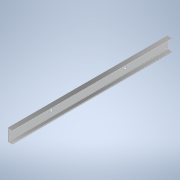
# Autodesk Inventor part: NASA-20-OP-01
Saved by Autodesk Inventor 2020 (Build 240168000, 168)
## iProperties
Created: 2019-09-07
Part Number: NASA-20-OP-01
Material: Aluminum 6061
Document SubType Name: Modeling
Designer: Rick Szalay
Density: 2.7 g/cm^3
Appearance: Aluminum - Flat
Author: Rick Szalay
Autodesk Inventor part; units mm, degrees
ref_plane "YZ Plane" through (0, 0, 0) normal (1, 0, 0) x (0, 1, 0)
ref_plane "XZ Plane" through (0, 0, 0) normal (0, 1, 0) x (-1, 0, 0)
ref_plane "XY Plane" through (0, 0, 0) normal (0, 0, 1) x (1, 0, 0)
sketch "Sketch1" plane through (0, 0, 0) normal (0, 0, 1) x (1, 0, 0)
  line L0 (0, 25.4) -> (0, -25.4)
  line L1 (0, -25.4) -> (19.05, -25.4)
  line L2 (0, 25.4) -> (19.05, 25.4)
  line L3 (19.05, 25.4) -> (19.05, 22.225)
  line L4 (19.05, 22.225) -> (3.048, 22.225)
  line L5 (3.048, 22.225) -> (3.048, -22.225)
  line L6 (3.048, -22.225) -> (19.05, -22.225)
  line L7 (19.05, -22.225) -> (19.05, -25.4)
  point P0 (0, 0)
  point P1 (0, 0)
  dimension "d0" = 50.8
  dimension "d1" = 19.05
  dimension "d2" = 3.175
  dimension "d3" = 16.002
  constraints: 16 end point, 5 perpendicular, 2 equal length, 2 vertical, 1 coincident, 1 horizontal, 1 midpoint, 1 point on line
  measures "d0" distance of L0.start L0.end
  measures "d1" distance of L0.start L2.end
  measures "d2" distance between parallel lines of L4 L2
  measures "d3" distance between parallel lines of L5 L7
extrude "Extrusion1" add sketch "Sketch1" along normal mid plane 660.4
fillet "Fillet1" radius 1.5875 4 edges at (3.048, 22.225, 0) (3.048, -22.225, 0) (19.05, -22.225, 0) (19.05, 22.225, 0)
sketch "Sketch2" plane through (3.048, -20.6375, -330.2) normal (1, 0, 0) x (0, 0, -1)
  point P0 (-330.2, 20.6375)
  point P1 (-177.8, 20.6375)
  point P2 (-482.6, 20.6375)
  dimension "d7" = 304.8
  dimension "d8" = 152.4
  constraints: 2 horizontal alignment
  measures "d7" distance of point (-482.6, 20.637) point (-177.8, 20.637)
  measures "d8" distance of point (-177.8, 20.637) point (-330.2, 20.637)
hole "Hole1" at (3.048, 0, -152.4) at (3.048, 0, 152.4) direction (-1, 0, 0) diameter 9.525 depth 25.4 tip angle 118
sketch "Sketch3" plane through (3.048, -20.6375, -330.2) normal (1, 0, 0) x (0, 0, -1)
  line L0 (-650.875, 33.3375) -> (-9.525, 33.3375)
  line L1 (-9.525, 33.3375) -> (-9.525, 7.9375)
  line L2 (-9.525, 7.9375) -> (-650.875, 7.9375)
  line L3 (-650.875, 7.9375) -> (-650.875, 33.3375)
  line L4 (-650.875, 33.3375) -> (-9.525, 7.9375) construction
  line L5 (-9.525, 33.3375) -> (-650.875, 7.9375) construction
  line L6 (0, 41.275) -> (0, 0) projected
  line L7 (-660.4, 0) -> (-660.4, 41.275) projected
  line L8 (0, -4.7625) -> (-660.4, -4.7625) projected
  line L9 (0, 46.0375) -> (-660.4, 46.0375) projected
  point P0 (-330.2, 20.6375)
  point P1 (-330.2, 7.9375)
  point P2 (-330.2, 33.3375)
  dimension "d34" = 9.525
  dimension "d35" = 9.525
  dimension "d36" = 12.7
  dimension "d37" = 12.7
  constraints: 12 end point, 4 coincident, 4 midpoint, 2 parallel, 1 horizontal, 1 perpendicular
  measures "d34" distance between parallel lines of L6 L1
  measures "d35" distance between parallel lines of L7 L3
  measures "d36" distance between parallel lines of L8 L2
  measures "d37" distance between parallel lines of L9 L0
hole "Hole2" at (3.048, -12.7, 320.675) at (3.048, 12.7, 320.675) at (3.048, -12.7, 0) at (3.048, 12.7, 0) at (3.048, -12.7, -320.675) at (3.048, 12.7, -320.675) direction (-1, 0, 0) diameter 5.1054 depth 25.4 tip angle 118 clearance for "Flat Head Machine Screw (82)" size "#10" standard "Ansi Unified Screw Threads"
sketch "Sketch5" plane through (3.048, -20.6375, -330.2) normal (1, 0, 0) x (0, 0, -1)
  circle A0 centre (-482.6, 20.6375) radius 4.7625 projected
  circle A1 centre (-177.8, 20.6375) radius 4.7625 projected
  point P0 (-330.2, 20.6375)
  point P1 (-466.6, 20.6375)
  point P2 (-498.6, 20.6375)
  point P3 (-193.8, 20.6375)
  point P4 (-161.8, 20.6375)
  dimension "d23" = 32
  dimension "d24" = 16
  dimension "d25" = 32
  dimension "d26" = 16
  constraints: 4 horizontal alignment
  measures "d23" distance of point (-466.6, 20.637) point (-498.6, 20.637)
  measures "d24" distance of point (-466.6, 20.637) A0.centre
  measures "d25" distance of point (-161.8, 20.637) point (-193.8, 20.637)
  measures "d26" distance of point (-193.8, 20.637) A1.centre
hole "Hole3" at (3.048, 0, 168.4) at (3.048, 0, 136.4) at (3.048, 0, -136.4) at (3.048, 0, -168.4) direction (-1, 0, 0) diameter 4.4958 end through all clearance for "Socket Head Cap Screw DIN EN ISO 4762" size "M4" standard "DIN"
equation "\"d4\" = Length"
equation "\"Length\" = 660.4"
body "Solid1"
